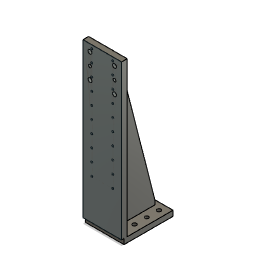
AAB400M (Autodesk Fusion 360 design; units mm, degrees)
Autodesk Fusion 360 part; units mm, degrees
sketch "Sketch2" plane through (0, 0, 0) normal (1, 0, 0) x (0, 0, -1)
  line L0 (0, 0) -> (140, 0)
  line L1 (140, 0) -> (140, 15)
  line L2 (140, 15) -> (0, 15)
  line L3 (0, 15) -> (0, 0)
  line L4 (9, 15) -> (-7, 15)
  line L5 (-7, 15) -> (-7, 455)
  line L6 (-7, 455) -> (9, 455)
  line L7 (9, 455) -> (9, 15)
  dimension "d1" = 16
  dimension "d2" = 15
  dimension "d3" = 140
  dimension "d4" = 7
  dimension "d5" = 455
  constraint horizontal L0
  constraint vertical L1
  constraint horizontal L2
  constraint vertical L3
  constraint coincident L0.start L3.end
  constraint horizontal L4
  constraint vertical L5
  constraint horizontal L6
  constraint vertical L7
  constraint coincident L2 L4.start
  measures "d1" distance of L5.end L6.end
  measures "d2" distance of L0.end L1.end
  measures "d3" distance of L1.end L2.end
  measures "d4" distance of L3 L5
  measures "d5" distance of L0 L6
extrude "Extrude1" add sketch "Sketch2" along normal mid plane 110
sketch "Sketch3" plane through (0, 0, 0) normal (1, 0, 0) x (0, 0, -1)
  line L0 (9, 15) -> (9, 455)
  line L1 (140, 15) -> (9, 15)
  line L2 (9, 442.5) -> (21, 442.5)
  line L3 (21, 442.5) -> (127.5, 27)
  line L4 (127.5, 27) -> (127.5, 15)
  dimension "d12" = 12
  dimension "d13" = 12.5
  dimension "d14" = 12.5
  dimension "d15" = 12
  constraint coincident L0 L2.start
  constraint perpendicular L0 L2
  constraint coincident L1 L4.end
  constraint perpendicular L1 L4
  measures "d12" distance of L2.start L2.end
  measures "d13" distance of L1.start L4
  measures "d14" distance of L0.end L2
  measures "d15" distance of L3.end L4.end
extrude "Extrude2" add sketch "Sketch3" along normal mid plane 31.76
sketch "Sketch4" plane through (0, 0, -9) normal (0, 0, -1) x (-1, 0, 0)
  line L0 (-15.88, 15) -> (-15.88, 442.5)
  line L1 (-15.88, 442.5) -> (15.88, 442.5)
  line L2 (15.88, 442.5) -> (15.88, 15)
  line L3 (15.88, 15) -> (55, 15)
  line L4 (55, 15) -> (55, 455)
  line L5 (55, 455) -> (-55, 455)
  line L6 (-55, 455) -> (-55, 15)
  line L7 (-55, 15) -> (-15.88, 15)
  line L8 (0, 455) -> (0, 0) construction
  circle A0 centre (-30, 445) radius 2.5
  circle A1 centre (-30, 410) radius 2.5
  circle A2 centre (-30, 375) radius 2.5
  circle A3 centre (-30, 340) radius 2.5
  circle A4 centre (-30, 305) radius 2.5
  circle A5 centre (-30, 270) radius 2.5
  circle A6 centre (-30, 235) radius 2.5
  circle A7 centre (-30, 200) radius 2.5
  circle A8 centre (-30, 165) radius 2.5
  circle A9 centre (-30, 130) radius 2.5
  circle A10 centre (30, 410) radius 2.5
  circle A11 centre (30, 375) radius 2.5
  circle A12 centre (30, 340) radius 2.5
  circle A13 centre (30, 305) radius 2.5
  circle A14 centre (30, 270) radius 2.5
  circle A15 centre (30, 235) radius 2.5
  circle A16 centre (30, 200) radius 2.5
  circle A17 centre (30, 165) radius 2.5
  circle A18 centre (30, 130) radius 2.5
  circle A19 centre (30, 445) radius 2.5
  dimension "d18" = 30
  dimension "d19" = 5
  dimension "d20" = 10
  dimension "d23" = 35
  dimension "d24" = 0
  constraint midpoint L5 L8.start
  constraint coincident L8.end origin
  constraint symmetric L8 A0 A19
  constraint symmetric L8 A1 A10
  constraint symmetric L8 A2 A11
  constraint symmetric L8 A3 A12
  constraint symmetric L8 A4 A13
  constraint symmetric L8 A5 A14
  constraint symmetric L8 A6 A15
  constraint symmetric L8 A7 A16
  constraint symmetric L8 A8 A17
  constraint symmetric L8 A9 A18
  measures "d18" distance of L8 A0.centre
  measures "d19" diameter of A0
  measures "d20" distance of L5 A0.centre
extrude "Extrude3" cut sketch "Sketch4" against normal blind 100 contours A0 | A1 | A2 | A3 | A4 | A5 | A6 | A7 | A8 | A9 | A10 | A11 | A12 | A13 | A14 | A15 | A16 | A17 | A18 | A19
sketch "Sketch5" plane through (0, 15, 0) normal (0, 1, 0) x (-1, 0, 0)
  line L0 (-15.88, -127.5) -> (-15.88, -9)
  line L1 (-15.88, -9) -> (-55, -9)
  line L2 (-55, -9) -> (-55, -140)
  line L3 (-55, -140) -> (55, -140)
  line L4 (55, -140) -> (55, -9)
  line L5 (55, -9) -> (15.88, -9)
  line L6 (15.88, -9) -> (15.88, -127.5)
  line L7 (15.88, -127.5) -> (-15.88, -127.5)
  circle A0 centre (37, -125) radius 3.9688
  circle A1 centre (37, -95) radius 3.9688
  circle A2 centre (37, -65) radius 3.9688
  circle A3 centre (37, -35) radius 3.9688
  line L8 (37, -125) -> (37, -35) construction
  line L9 (37, -80) -> (52, -80) construction
  line L10 (52, -80) -> (52, -75.9045) construction
  circle A4 centre (67, -125) radius 3.9688
  circle A5 centre (67, -95) radius 3.9688
  circle A6 centre (67, -65) radius 3.9688
  circle A7 centre (67, -35) radius 3.9688
  line L11 (0, -140) -> (0, 0) construction
  line L12 (-52, -80) -> (-52, -75.9045) construction
  circle A8 centre (-67, -95) radius 3.9688
  line L13 (-37, -80) -> (-52, -80) construction
  circle A9 centre (-67, -125) radius 3.9688
  circle A10 centre (-37, -95) radius 3.9688
  circle A11 centre (-37, -65) radius 3.9688
  circle A12 centre (-67, -65) radius 3.9688
  circle A13 centre (-67, -35) radius 3.9688
  circle A14 centre (-37, -35) radius 3.9688
  line L14 (-37, -125) -> (-37, -35) construction
  circle A15 centre (-37, -125) radius 3.9688
  dimension "d27" = 7.9375
  dimension "d28" = 37
  dimension "d29" = 125
  dimension "d30" = 30
  dimension "d31" = 30
  dimension "d32" = 30
  dimension "d33" = 30
  constraint equal A2 A3
  constraint equal A1 A2
  constraint equal A0 A1
  constraint coincident A0.centre L8.start
  constraint coincident A3.centre L8.end
  constraint coincident A2.centre L8
  constraint vertical L8
  constraint coincident A1.centre L8
  constraint midpoint L8 L9.start
  constraint perpendicular L8 L9
  constraint perpendicular L9 L10
  constraint symmetric A0 L10 A4
  constraint symmetric A1 L10 A5
  constraint symmetric A2 L10 A6
  constraint symmetric A3 L10 A7
  constraint midpoint L3 L11.start
  constraint coincident L11.end origin
  constraint symmetric A0 L11 A15
  constraint symmetric A1 L11 A10
  constraint symmetric A2 L11 A11
  constraint symmetric A3 L11 A14
  constraint symmetric A0.centre L11 L14.start
  constraint symmetric A3.centre L11 A14.centre
  constraint symmetric L9.start L11 L13.start
  constraint symmetric L9.end L11 L12.start
  constraint symmetric L10.end L11 L12.end
  constraint symmetric A4 L11 A9
  constraint symmetric A5 L11 A8
  constraint symmetric A6 L11 A12
  constraint symmetric A7 L11 A13
  measures "d27" diameter of A3
  measures "d28" distance of L11.end L8
  measures "d29" vertical distance of L11.end A0.centre
  measures "d30" distance of A0.centre A1.centre
  measures "d31" distance of A1.centre A2.centre
  measures "d32" distance of A2.centre A3.centre
  measures "d33" distance of A2.centre A6.centre
sketch "Sketch6" plane through (0, 0, 7) normal (0, 0, 1) x (1, 0, 0)
  circle A0 centre (30, 235) radius 2.5
  circle A1 centre (-30, 200) radius 2.5
  circle A2 centre (30, 270) radius 2.5
  circle A3 centre (-30, 340) radius 2.5
  circle A4 centre (30, 410) radius 2.5
  circle A5 centre (-30, 445) radius 2.5
  circle A6 centre (30, 375) radius 2.5
  circle A7 centre (-30, 270) radius 2.5
  circle A8 centre (-30, 165) radius 2.5
  circle A9 centre (30, 130) radius 2.5
  circle A10 centre (30, 200) radius 2.5
  circle A11 centre (-30, 235) radius 2.5
  circle A12 centre (30, 305) radius 2.5
  circle A13 centre (-30, 375) radius 2.5
  circle A14 centre (30, 445) radius 2.5
  circle A15 centre (-30, 410) radius 2.5
  circle A16 centre (30, 340) radius 2.5
  circle A17 centre (-30, 305) radius 2.5
  circle A18 centre (30, 165) radius 2.5
  circle A19 centre (-30, 130) radius 2.5
  line L0 (-55, 15) -> (55, 15)
  line L1 (55, 15) -> (55, 455)
  line L2 (55, 455) -> (-55, 455)
  line L3 (-55, 455) -> (-55, 15)
sketch "Sketch7" plane through (0, 0, 0) normal (0, -1, 0) x (1, 0, 0)
  line L0 (-55, -140) -> (55, -140)
  line L1 (55, -140) -> (55, 0)
  line L2 (55, 0) -> (-55, 0)
  line L3 (-55, 0) -> (-55, -140)
  circle A0 centre (-35, -120) radius 5.5
  circle A1 centre (35, -120) radius 5.5
  circle A2 centre (-35, -85) radius 5
  circle A3 centre (35, -85) radius 5
  circle A4 centre (-35, -50) radius 5.5
  circle A5 centre (35, -50) radius 5.5
  dimension "d36" = 20
  dimension "d37" = 20
  dimension "d38" = 11
  dimension "d39" = 35
  dimension "d40" = 10
  dimension "d41" = 70
  dimension "d42" = 20
  dimension "d43" = 35
  constraint equal A0 A1
  constraint vertical A0.centre A2.centre
  constraint horizontal A2.centre A3.centre
  constraint vertical A1.centre A3.centre
  constraint equal A2 A3
  constraint vertical A2.centre A4.centre
  constraint vertical A3.centre A5.centre
  constraint horizontal A4.centre A5.centre
  constraint equal A4 A5
  constraint equal A0 A5
  measures "d36" distance of L0 A0.centre
  measures "d37" distance of L3 A0.centre
  measures "d38" diameter of A0
  measures "d39" vertical distance of A0.centre A2.centre
  measures "d40" diameter of A2
  measures "d41" horizontal distance of A0.centre A1.centre
  measures "d42" distance of L0 A1.centre
  measures "d43" distance of A2.centre A4.centre
extrude "Extrude5" cut sketch "Sketch7" against normal blind 35 contours A0 | A1 | A2 | A3 | A4 | A5
sketch "Sketch8" plane through (0, 0, 7) normal (0, 0, 1) x (1, 0, 0)
  circle A0 centre (-35, 400) radius 4
  circle A1 centre (35, 400) radius 4
  line L0 (55, 15) -> (55, 455)
  line L1 (-55, 455) -> (-55, 15)
  circle A2 centre (-35, 435) radius 5.5
  circle A3 centre (35, 435) radius 5.5
  circle A4 centre (-35, 365) radius 5.5
  circle A5 centre (35, 365) radius 5.5
  dimension "d46" = 400
  dimension "d47" = 20
  dimension "d48" = 20
  dimension "d49" = 8
  dimension "d50" = 35
  dimension "d51" = 35
  dimension "d52" = 11
  dimension "d53" = 35
  dimension "d54" = 35
  constraint horizontal A0.centre A1.centre
  constraint equal A0 A1
  constraint vertical A0.centre A2.centre
  constraint vertical A1.centre A3.centre
  constraint equal A2 A3
  constraint equal A4 A5
  constraint vertical A0.centre A4.centre
  constraint vertical A1.centre A5.centre
  constraint equal A3 A4
  measures "d46" vertical distance of origin A0.centre
  measures "d47" distance of A1.centre L0
  measures "d48" distance of A0.centre L1
  measures "d49" diameter of A0
  measures "d50" distance of A0.centre A2.centre
  measures "d51" distance of A1.centre A3.centre
  measures "d52" diameter of A3
  measures "d53" distance of A0.centre A4.centre
  measures "d54" distance of A1.centre A5.centre
extrude "Extrude6" cut sketch "Sketch8" against normal blind 60
equation "d27 = 5 / 16 * 1 in"
